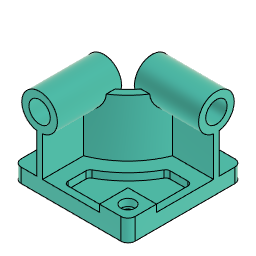
Exercise-9 v1 (Autodesk Fusion 360 design; units mm, degrees)
Autodesk Fusion 360 part; units mm, degrees
note: some values were not read from the file. Set by a fixed rule: which sketch regions a step uses.
sketch "Sketch1" plane through (0, 0, 0) normal (0, 0, 1) x (1, 0, 0)
  line L0 (20, -20) -> (-20, -20)
  line L1 (-20, -20) -> (-20, 20)
  line L2 (-20, 20) -> (20, 20)
  line L3 (20, 20) -> (20, -20)
  line L4 (-20, -20) -> (20, 20) construction
  line L5 (20, -20) -> (10, -20)
  line L6 (10, -20) -> (10, -10)
  line L7 (10, -10) -> (20, -10)
  line L8 (20, -10) -> (20, -20)
  line L9 (-12, -20) -> (-12, -3.6854)
  line L10 (3.6854, 12) -> (20, 12)
  line L11 (-10, -20) -> (-10, -5.6174)
  line L12 (5.6174, 10) -> (20, 10)
  arc A0 (-10, -5.6174) -> (5.6174, 10) centre (-20, 20) ccw
  arc A1 (-12, -3.6854) -> (3.6854, 12) centre (-20, 20) ccw
  line L13 (20, -20) -> (-2.3223, 2.3223) construction
  line L14 (-10, 10) -> (-20, 20) construction
  line L15 (17.5, 5) -> (17.5, -10)
  line L16 (10, -17.5) -> (-5, -17.5)
  line L17 (-5, -17.5) -> (-5, -8.8314)
  arc A2 (-5, -8.8314) -> (8.8314, 5) centre (-20, 20) ccw
  line L18 (8.8314, 5) -> (17.5, 5)
  circle A3 centre (15, -15) radius 2.5
  circle A4 centre (15, -15) radius 1.5
  dimension "d1" = 40
  dimension "d2" = 40
  dimension "d3" = 10
  dimension "d4" = 10
  dimension "d5" = 50
  dimension "d6" = 55
  dimension "d7" = 8
  dimension "d9" = 2.5
  dimension "d10" = 2.5
  dimension "d12" = 5
  dimension "d13" = 3
  dimension "d14" = 5
  constraint horizontal L0
  constraint perpendicular L0 L1
  constraint parallel L0 L2
  constraint parallel L1 L3
  constraint coincident origin L13
  constraint coincident L4 origin
  constraint horizontal L5
  constraint vertical L6
  constraint horizontal L7
  constraint vertical L8
  constraint coincident L1.end L2.start
  constraint concentric A0 A1
  constraint coincident L0 L9.start
  constraint perpendicular L0 L9
  constraint coincident L3 L10.end
  constraint perpendicular L3 L10
  constraint coincident A1 L13.end
  constraint collinear L13 L14
  constraint perpendicular L12 L15
  constraint coincident L7 L15.end
  constraint coincident L6 L16.start
  constraint perpendicular L11 L16
  constraint coincident L13 A3.centre
  constraint concentric A3 A4
  constraint concentric A0 A2
  measures "d1" distance of L1.end L2.end
  measures "d2" distance of L0.end L1.end
  measures "d3" distance of L0.start L5.end
  measures "d4" distance of L0.start L7.end
  measures "d5" diameter of A1
  measures "d6" diameter of A0
  measures "d7" distance of L2 L10
  measures "d9" distance of L0 L16
  measures "d10" distance of L3 L15
  measures "d12" diameter of A3
  measures "d13" diameter of A4
  measures "d14" distance of L6 A3.centre
extrude "Extrude1" add sketch "Sketch1" against normal blind 5 contours L0 L3 L5 L6 L7 L8 | L0 L3 L6 L7 L11 L12 A0 L15 L16 L17 A2 L18 | L0 L3 L9 L10 L11 L12 A0 A1 | L6 L7 L15 L16 L17 A2 L18 | L0 L1 L2 L3 L9 L10 A1 | A3 | A4
extrude "Extrude2" cut sketch "Sketch1" against normal blind 2.5 contours L6 L7 L15 L16 L17 A2 L18
extrude "Extrude3" cut sketch "Sketch1" against normal blind 17 contours A4
extrude "Extrude4" add sketch "Sketch1" along normal blind 2.5 contours L0 L3 L5 L6 L7 L8
extrude "Extrude5" add sketch "Sketch1" along normal blind 20 contours L0 L3 L9 L10 L11 L12 A0 A1
fillet "Fillet1" radius 2.5 4 edges at (20, -20, -1.25) (20, 20, -2.5) (-20, -20, -2.5) (-20, 20, -2.5)
fillet "Fillet2" radius 1.5 4 edges at (-5, -8.8314, -1.25) (8.8314, 5, -1.25) (-5, -17.5, -1.25) (17.5, 5, -1.25)
sketch "Sketch2" plane through (0, -20, 0) normal (0, -1, 0) x (1, 0, 0)
  line L0 (-17.5, 0) -> (-17.5, -5)
  line L1 (-17.5, -5) -> (17.5, -5)
  line L2 (17.5, -5) -> (17.5, 2.5)
  line L3 (17.5, 2.5) -> (10, 2.5)
  line L4 (10, 2.5) -> (10, 0)
  line L5 (10, 0) -> (-10, 0)
  line L6 (-10, 0) -> (-10, 20)
  line L7 (-10, 20) -> (-12, 20)
  line L8 (-12, 20) -> (-12, 0)
  line L9 (-12, 0) -> (-17.5, 0)
  circle A0 centre (-11, 20) radius 6.25
  dimension "d29" = 12.5
  constraint midpoint L7 A0.centre
  measures "d29" diameter of A0
extrude "Extrude6" add sketch "Sketch2" against normal blind 22.5 contours L6 L7 L8 A0 | L6 L7 L8 A0
sketch "Sketch3" plane through (20, 0, 0) normal (1, 0, 0) x (0, 1, 0)
  line L0 (17.5, -5) -> (17.5, 0)
  line L1 (17.5, 0) -> (12, 0)
  line L2 (12, 0) -> (12, 20)
  line L3 (12, 20) -> (10, 20)
  line L4 (10, 20) -> (10, 0)
  line L5 (10, 0) -> (-10, 0)
  line L6 (-10, 0) -> (-10, 2.5)
  line L7 (-10, 2.5) -> (-17.5, 2.5)
  line L8 (-17.5, 2.5) -> (-17.5, -5)
  line L9 (-17.5, -5) -> (17.5, -5)
  circle A0 centre (11, 20) radius 6.25
  dimension "d32" = 12.5
  constraint midpoint L3 A0.centre
  measures "d32" diameter of A0
extrude "Extrude7" add sketch "Sketch3" against normal blind 22.5 contours L2 L3 L4 A0 | L2 L3 L4 A0
hole "Hole1" at (-11, -20, 20) direction (0, 1, 0) diameter 7.5 end through all
hole "Hole2" at (20, 11, 20) direction (-1, 0, 0) diameter 7.5 end through all
